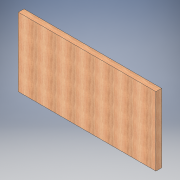
# Autodesk Inventor part: rev2 top large wall plane
Saved by Autodesk Inventor 2017 (Build 210142000, 142)
## iProperties
Created: 2019-05-04
Part Number: rev2 top large wall plane
Material: Wood (Birch)
Document SubType Name: Modeling
Designer: Roman
Density: 0.55 g/cm^3
Appearance: Birch - Natural Polished
Author: Roman
Autodesk Inventor part; units mm, degrees
ref_plane "YZ Plane" through (0, 0, 0) normal (1, 0, 0) x (0, 1, 0)
ref_plane "XZ Plane" through (0, 0, 0) normal (0, 1, 0) x (-1, 0, 0)
ref_plane "XY Plane" through (0, 0, 0) normal (0, 0, 1) x (1, 0, 0)
sketch "Sketch2" plane through (0, 0, 0) normal (0, 1, 0) x (-1, 0, 0)
  line L0 (0, 0) -> (-1828.8, 0)
  line L1 (-1828.8, 0) -> (-1828.8, -76.2)
  line L2 (-1828.8, -76.2) -> (0, -76.2)
  line L3 (0, -76.2) -> (0, 0)
  dimension "d4" = 1828.8
  dimension "d5" = 76.2
  constraints: 8 end point, 2 parallel, 1 horizontal, 1 perpendicular
  measures "d4" distance of L2.end L1.end
  measures "d5" distance of L1.end L0.end
extrude "Extrusion2" add sketch "Sketch2" along normal blind 914.4
body "Solid2"
